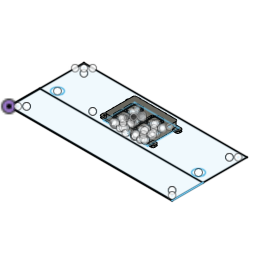
rockclimbingwall v6 (Autodesk Fusion 360 design; units mm, degrees)
Autodesk Fusion 360 part; units mm, degrees
note: some values were not read from the file. Set by a fixed rule: which sketch regions a step uses.
(part 1 of 4)
sketch "Sketch1" plane through (0, 0, 0) normal (0, 0, 1) x (1, 0, 0)
  line L0 (0, 0) -> (469.9, 0)
  line L1 (469.9, 0) -> (469.9, 215.9)
  line L2 (469.9, 215.9) -> (0, 215.9)
  line L3 (0, 215.9) -> (0, 0)
  line L4 (0, 0) -> (469.9, 0)
  line L5 (469.9, 0) -> (469.9, 88.9)
  line L6 (469.9, 88.9) -> (0, 88.9)
  line L7 (0, 88.9) -> (0, 0)
  circle A0 centre (31.75, 107.95) radius 13.97
  circle A1 centre (438.15, 107.95) radius 13.97
  circle A2 centre (234.95, 107.95) radius 3.175
  line L8 (195.58, 163.3039) -> (195.58, 144.036)
  line L9 (215.9, 144.0361) -> (215.9, 163.3039)
  line L10 (197.3761, 165.1) -> (214.104, 165.1)
  line L11 (214.104, 142.24) -> (197.3761, 142.24)
  line L12 (223.52, 163.304) -> (223.52, 144.0362)
  line L13 (187.96, 144.036) -> (187.96, 163.3039)
  line L14 (214.104, 172.72) -> (197.3761, 172.72)
  line L15 (197.3761, 134.62) -> (214.104, 134.62)
  line L16 (193.938, 168.012) -> (196.478, 165.472)
  line L17 (192.668, 166.742) -> (195.208, 164.202)
  line L18 (215.002, 165.472) -> (217.542, 168.012)
  line L19 (216.272, 164.202) -> (218.812, 166.742)
  line L20 (215.002, 172.348) -> (217.542, 169.808)
  line L21 (223.148, 164.202) -> (220.608, 166.742)
  line L22 (196.478, 172.348) -> (193.938, 169.808)
  line L23 (190.872, 166.742) -> (188.332, 164.202)
  line L24 (190.872, 140.598) -> (188.332, 143.138)
  line L25 (196.478, 134.992) -> (193.938, 137.532)
  line L26 (220.608, 140.5981) -> (223.148, 143.1381)
  line L27 (215.002, 134.992) -> (217.542, 137.532)
  line L28 (195.208, 143.138) -> (192.668, 140.598)
  line L29 (196.478, 141.868) -> (193.938, 139.328)
  line L30 (195.58, 163.83) -> (195.58, 163.83)
  line L31 (192.668, 166.742) -> (195.208, 164.202) construction
  line L32 (216.272, 143.1381) -> (218.8119, 140.5981) construction
  line L33 (214.63, 162.56) -> (214.63, 162.56)
  line L34 (218.812, 166.742) -> (216.272, 164.202) construction
  line L35 (195.208, 143.138) -> (192.668, 140.598) construction
  line L36 (216.272, 143.1381) -> (218.8119, 140.5981)
  line L37 (215.002, 141.868) -> (217.542, 139.328)
  arc A3 (197.3761, 172.72) -> (196.478, 172.348) centre (197.3761, 171.45) ccw
  arc A4 (193.938, 169.808) -> (193.938, 168.012) centre (194.8361, 168.91) ccw
  arc A5 (196.478, 165.472) -> (197.3761, 165.1) centre (197.3761, 166.37) ccw
  arc A6 (215.002, 172.348) -> (214.104, 172.72) centre (214.104, 171.45) ccw
  arc A7 (217.542, 168.012) -> (217.542, 169.808) centre (216.644, 168.91) ccw
  arc A8 (214.104, 165.1) -> (215.002, 165.472) centre (214.104, 166.37) ccw
  arc A9 (192.668, 166.742) -> (190.872, 166.742) centre (191.77, 165.844) ccw
  arc A10 (195.58, 163.3039) -> (195.208, 164.202) centre (194.31, 163.3039) ccw
  arc A11 (188.332, 164.202) -> (187.96, 163.3039) centre (189.23, 163.3039) ccw
  arc A12 (187.96, 144.036) -> (188.332, 143.138) centre (189.23, 144.036) ccw
  arc A13 (190.872, 140.598) -> (192.668, 140.598) centre (191.77, 141.496) ccw
  arc A14 (195.208, 143.138) -> (195.58, 144.036) centre (194.31, 144.036) ccw
  arc A15 (218.8119, 140.5981) -> (220.608, 140.5981) centre (219.71, 141.4962) ccw
  arc A16 (215.9, 144.0361) -> (216.272, 143.1381) centre (217.17, 144.0361) ccw
  arc A17 (223.148, 143.1381) -> (223.52, 144.0362) centre (222.25, 144.0362) ccw
  arc A18 (220.608, 166.742) -> (218.812, 166.742) centre (219.71, 165.8439) ccw
  arc A19 (223.52, 163.304) -> (223.148, 164.202) centre (222.25, 163.304) ccw
  arc A20 (216.272, 164.202) -> (215.9, 163.3039) centre (217.17, 163.3039) ccw
  arc A21 (193.938, 139.328) -> (193.938, 137.532) centre (194.8361, 138.43) ccw
  arc A22 (197.3761, 142.24) -> (196.478, 141.868) centre (197.3761, 140.97) ccw
  arc A23 (196.478, 134.992) -> (197.3761, 134.62) centre (197.3761, 135.89) ccw
  arc A24 (214.104, 134.62) -> (215.002, 134.992) centre (214.104, 135.89) ccw
  arc A25 (217.542, 137.532) -> (217.542, 139.328) centre (216.644, 138.43) ccw
  arc A26 (215.002, 141.868) -> (214.104, 142.24) centre (214.104, 140.97) ccw
  line L38 (223.148, 112.658) -> (220.608, 110.118)
  line L39 (190.872, 110.118) -> (188.332, 112.658)
  line L40 (215.002, 104.512) -> (217.542, 107.052)
  line L41 (223.52, 113.556) -> (223.52, 132.8238)
  line L42 (218.812, 110.118) -> (218.44, 110.49) construction
  line L43 (192.668, 110.118) -> (195.208, 112.658) construction
  line L44 (192.668, 110.118) -> (195.208, 112.658)
  line L45 (216.272, 112.658) -> (218.812, 110.118)
  line L46 (215.002, 111.388) -> (217.542, 108.848)
  line L47 (215.9, 132.8239) -> (215.9, 113.5561)
  line L48 (193.938, 108.848) -> (196.478, 111.388)
  arc A27 (195.208, 112.658) -> (195.58, 113.5561) centre (194.31, 113.5561) ccw
  line L49 (214.63, 114.3) -> (214.63, 114.3)
  arc A28 (214.104, 104.14) -> (215.002, 104.512) centre (214.104, 105.41) ccw
  arc A29 (190.872, 110.118) -> (192.668, 110.118) centre (191.77, 111.016) ccw
  line L50 (187.96, 132.824) -> (187.96, 113.5561)
  line L51 (197.3761, 111.76) -> (214.104, 111.76)
  line L52 (214.104, 104.14) -> (197.3761, 104.14)
  line L53 (195.58, 113.5561) -> (195.58, 132.824)
  arc A30 (223.148, 112.658) -> (223.52, 113.556) centre (222.25, 113.556) ccw
  arc A31 (215.002, 111.388) -> (214.104, 111.76) centre (214.104, 110.49) ccw
  line L54 (195.58, 113.03) -> (195.58, 113.03)
  arc A32 (196.478, 104.512) -> (197.3761, 104.14) centre (197.3761, 105.41) ccw
  arc A33 (197.3761, 111.76) -> (196.478, 111.388) centre (197.3761, 110.49) ccw
  arc A34 (215.9, 113.5561) -> (216.272, 112.658) centre (217.17, 113.5561) ccw
  line L55 (196.478, 104.512) -> (193.938, 107.052)
  arc A35 (195.58, 132.824) -> (195.208, 133.722) centre (194.31, 132.824) ccw
  arc A36 (218.812, 110.118) -> (220.608, 110.118) centre (219.71, 111.0161) ccw
  arc A37 (193.938, 108.848) -> (193.938, 107.052) centre (194.8361, 107.95) ccw
  arc A38 (187.96, 113.5561) -> (188.332, 112.658) centre (189.23, 113.5561) ccw
  arc A39 (192.668, 136.262) -> (190.872, 136.262) centre (191.77, 135.364) ccw
  line L56 (195.208, 133.722) -> (192.668, 136.262) construction
  arc A40 (223.52, 132.8238) -> (223.148, 133.7219) centre (222.25, 132.8238) ccw
  arc A41 (188.332, 133.722) -> (187.96, 132.824) centre (189.23, 132.824) ccw
  line L57 (220.608, 136.2619) -> (223.148, 133.7219)
  arc A42 (216.272, 133.7219) -> (215.9, 132.8239) centre (217.17, 132.8239) ccw
  arc A43 (220.608, 136.2619) -> (218.8119, 136.2619) centre (219.71, 135.3638) ccw
  line L58 (195.208, 133.722) -> (192.668, 136.262)
  line L59 (216.272, 133.7219) -> (218.8119, 136.2619)
  line L60 (190.872, 136.262) -> (188.332, 133.722)
  line L61 (216.272, 133.7219) -> (218.8119, 136.2619) construction
  arc A44 (217.542, 107.052) -> (217.542, 108.848) centre (216.644, 107.95) ccw
  line L62 (249.292, 136.2619) -> (246.752, 133.7219)
  arc A45 (254.898, 134.992) -> (255.796, 134.62) centre (255.796, 135.89) ccw
  line L63 (254.898, 104.512) -> (252.358, 107.052)
  line L64 (273.422, 104.512) -> (275.962, 107.052)
  line L65 (246.752, 112.658) -> (249.292, 110.118)
  line L66 (281.94, 132.824) -> (281.94, 113.5561)
  line L67 (246.38, 113.556) -> (246.38, 132.8238)
  line L68 (255.796, 104.14) -> (272.5239, 104.14)
  line L69 (279.028, 110.118) -> (281.568, 112.658)
  arc A46 (252.358, 108.848) -> (252.358, 107.052) centre (253.256, 107.95) ccw
  line L70 (277.232, 110.118) -> (274.692, 112.658)
  line L71 (253.628, 164.202) -> (251.088, 166.742)
  arc A47 (253.628, 112.658) -> (254, 113.5561) centre (252.73, 113.5561) ccw
  line L72 (254.898, 165.472) -> (252.358, 168.012)
  line L73 (275.962, 108.848) -> (273.422, 111.388)
  line L74 (274.32, 113.03) -> (274.32, 113.03)
  line L75 (272.5239, 134.62) -> (255.796, 134.62)
  arc A48 (254.898, 104.512) -> (255.796, 104.14) centre (255.796, 105.41) ccw
  arc A49 (274.692, 133.722) -> (274.32, 132.824) centre (275.59, 132.824) ccw
  arc A50 (272.5239, 104.14) -> (273.422, 104.512) centre (272.5239, 105.41) ccw
  line L76 (251.088, 110.118) -> (253.628, 112.658) construction
  line L77 (277.232, 166.742) -> (274.692, 164.202) construction
  arc A51 (246.38, 113.556) -> (246.752, 112.658) centre (247.65, 113.556) ccw
  arc A52 (275.962, 107.052) -> (275.962, 108.848) centre (275.0639, 107.95) ccw
  arc A53 (277.232, 110.118) -> (279.028, 110.118) centre (278.13, 111.016) ccw
  line L78 (255.27, 114.3) -> (255.27, 114.3)
  line L79 (277.232, 166.742) -> (274.692, 164.202)
  arc A54 (274.32, 113.5561) -> (274.692, 112.658) centre (275.59, 113.5561) ccw
  line L80 (254, 132.8239) -> (254, 113.5561)
  arc A55 (281.94, 132.824) -> (281.568, 133.722) centre (280.67, 132.824) ccw
  line L81 (274.32, 113.5561) -> (274.32, 132.824)
  arc A56 (255.796, 111.76) -> (254.898, 111.388) centre (255.796, 110.49) ccw
  arc A57 (281.568, 112.658) -> (281.94, 113.5561) centre (280.67, 113.5561) ccw
  line L82 (253.628, 133.7219) -> (251.0881, 136.2619)
  line L83 (279.028, 136.262) -> (281.568, 133.722)
  line L84 (253.628, 133.7219) -> (251.0881, 136.2619) construction
  arc A58 (249.292, 110.118) -> (251.088, 110.118) centre (250.19, 111.0161) ccw
  line L85 (274.692, 133.722) -> (277.232, 136.262) construction
  line L86 (274.692, 133.722) -> (277.232, 136.262)
  arc A59 (246.752, 133.7219) -> (246.38, 132.8238) centre (247.65, 132.8238) ccw
  line L87 (254.898, 111.388) -> (252.358, 108.848)
  arc A60 (272.5239, 134.62) -> (273.422, 134.992) centre (272.5239, 135.89) ccw
  line L88 (253.628, 112.658) -> (251.088, 110.118)
  arc A61 (273.422, 111.388) -> (272.5239, 111.76) centre (272.5239, 110.49) ccw
  line L89 (251.088, 166.742) -> (253.628, 164.202) construction
  arc A62 (255.796, 172.72) -> (254.898, 172.348) centre (255.796, 171.45) ccw
  line L90 (255.27, 162.56) -> (255.27, 162.56)
  arc A63 (246.38, 144.0362) -> (246.752, 143.1381) centre (247.65, 144.0362) ccw
  line L91 (272.5239, 111.76) -> (255.796, 111.76)
  arc A64 (279.028, 166.742) -> (277.232, 166.742) centre (278.13, 165.844) ccw
  line L92 (274.32, 163.3039) -> (274.32, 144.036)
  line L93 (281.94, 144.036) -> (281.94, 163.3039)
  arc A65 (275.962, 168.012) -> (275.962, 169.808) centre (275.0639, 168.91) ccw
  line L94 (255.796, 172.72) -> (272.5239, 172.72)
  line L95 (253.628, 143.1381) -> (251.0881, 140.5981) construction
  line L96 (272.5239, 165.1) -> (255.796, 165.1)
  line L97 (277.232, 110.118) -> (274.692, 112.658) construction
  arc A66 (252.358, 169.808) -> (252.358, 168.012) centre (253.256, 168.91) ccw
  line L98 (246.752, 164.202) -> (249.292, 166.742)
  line L99 (254.898, 172.348) -> (252.358, 169.808)
  arc A67 (272.5239, 165.1) -> (273.422, 165.472) centre (272.5239, 166.37) ccw
  line L100 (246.38, 163.304) -> (246.38, 144.0362)
  line L101 (273.422, 141.868) -> (275.962, 139.328)
  line L102 (255.796, 142.24) -> (272.5239, 142.24)
  line L103 (279.028, 140.598) -> (281.568, 143.138)
  arc A68 (249.292, 140.5981) -> (251.0881, 140.5981) centre (250.19, 141.4962) ccw
  line L104 (273.422, 134.992) -> (275.962, 137.532)
  arc A69 (281.94, 163.3039) -> (281.568, 164.202) centre (280.67, 163.3039) ccw
  arc A70 (252.358, 139.328) -> (252.358, 137.532) centre (253.256, 138.43) ccw
  arc A71 (254, 163.3039) -> (253.628, 164.202) centre (252.73, 163.3039) ccw
  line L105 (274.32, 163.83) -> (274.32, 163.83)
  arc A72 (251.088, 166.742) -> (249.292, 166.742) centre (250.19, 165.8439) ccw
  line L106 (274.692, 143.138) -> (277.232, 140.598) construction
  line L107 (274.692, 143.138) -> (277.232, 140.598)
  line L108 (254.898, 141.868) -> (252.358, 139.328)
  line L109 (253.628, 143.1381) -> (251.0881, 140.5981)
  line L110 (273.422, 172.348) -> (275.962, 169.808)
  arc A73 (254.898, 165.472) -> (255.796, 165.1) centre (255.796, 166.37) ccw
  line L111 (275.962, 168.012) -> (273.422, 165.472)
  line L112 (279.028, 166.742) -> (281.568, 164.202)
  line L113 (254, 144.0361) -> (254, 163.3039)
  arc A74 (255.796, 142.24) -> (254.898, 141.868) centre (255.796, 140.97) ccw
  arc A75 (273.422, 172.348) -> (272.5239, 172.72) centre (272.5239, 171.45) ccw
  arc A76 (253.628, 143.1381) -> (254, 144.0361) centre (252.73, 144.0361) ccw
  line L114 (249.292, 140.5981) -> (246.752, 143.1381)
  arc A77 (246.752, 164.202) -> (246.38, 163.304) centre (247.65, 163.304) ccw
  line L115 (254.898, 134.992) -> (252.358, 137.532)
  arc A78 (275.962, 137.532) -> (275.962, 139.328) centre (275.0639, 138.43) ccw
  arc A79 (274.692, 164.202) -> (274.32, 163.3039) centre (275.59, 163.3039) ccw
  arc A80 (273.422, 141.868) -> (272.5239, 142.24) centre (272.5239, 140.97) ccw
  arc A81 (281.568, 143.138) -> (281.94, 144.036) centre (280.67, 144.036) ccw
  arc A82 (279.028, 136.262) -> (277.232, 136.262) centre (278.13, 135.364) ccw
  arc A83 (251.0881, 136.2619) -> (249.292, 136.2619) centre (250.19, 135.3638) ccw
  arc A84 (274.32, 144.036) -> (274.692, 143.138) centre (275.59, 144.036) ccw
  arc A85 (277.232, 140.598) -> (279.028, 140.598) centre (278.13, 141.496) ccw
  arc A86 (254, 132.8239) -> (253.628, 133.7219) centre (252.73, 132.8239) ccw
  line L116 (234.95, 101.6) -> (298.45, 101.6)
  line L117 (298.45, 101.6) -> (171.45, 101.6)
  line L118 (171.45, 101.6) -> (171.45, 190.5)
  line L119 (171.45, 190.5) -> (298.45, 190.5)
  line L120 (298.45, 190.5) -> (298.45, 101.6)
  circle A87 centre (189.23, 110.49) radius 1.5875
  circle A88 centre (281.94, 110.49) radius 1.5875
  circle A89 centre (281.94, 180.34) radius 1.5875
  circle A90 centre (189.23, 180.34) radius 1.5875
  circle A91 centre (133.35, 107.95) radius 3.175
  circle A92 centre (133.35, 107.95) radius 6.35
  line L121 (281.94, 113.5561) -> (281.94, 132.824)
  line L122 (281.94, 144.036) -> (281.94, 163.3039)
  line L123 (0, 215.9) -> (25.4, 215.9)
  line L124 (0, 190.5) -> (0, 215.9)
  circle A93 centre (25.4, 190.5) radius 6.35
  circle A94 centre (444.5, 190.5) radius 6.35
  circle A95 centre (25.4, 25.4) radius 6.35
  circle A96 centre (444.5, 25.4) radius 6.35
  circle A97 centre (25.4, 190.5) radius 4.1275
  line L125 (171.45, 190.5) -> (298.45, 190.5)
  circle A98 centre (444.5, 190.5) radius 4.1275
  circle A99 centre (444.5, 25.4) radius 4.1275
  circle A100 centre (25.4, 25.4) radius 4.1275
  circle A101 centre (12.7, 203.2) radius 0.635
  circle A102 centre (457.2, 203.2) radius 0.635
  circle A103 centre (457.2, 12.7) radius 0.635
  circle A104 centre (12.7, 12.7) radius 0.635
  point P0 (214.63, 165.1)
  point P1 (214.63, 142.24)
  point P2 (196.85, 142.24)
  point P3 (205.74, 153.67)
  point P4 (205.74, 153.67)
  point P5 (205.74, 153.67)
  point P6 (214.104, 134.62)
  point P7 (215.002, 134.992)
  point P8 (214.63, 111.76)
  point P9 (197.3761, 134.62)
  point P10 (214.63, 134.62)
  point P11 (196.478, 134.992)
  point P12 (191.77, 115.57)
  point P13 (213.36, 107.95)
  point P14 (214.104, 135.89)
  point P15 (219.71, 130.81)
  point P16 (219.71, 115.57)
  point P17 (197.3761, 135.89)
  point P18 (205.74, 123.19)
  point P19 (205.74, 123.19)
  point P20 (196.85, 134.62)
  point P21 (198.12, 107.95)
  point P22 (205.74, 123.19)
  point P23 (191.77, 130.81)
  point P24 (264.16, 153.67)
  point P25 (264.16, 123.19)
  point P26 (264.16, 123.19)
  point P27 (278.13, 130.81)
  point P28 (255.796, 135.89)
  point P29 (254.898, 134.992)
  point P30 (273.422, 134.992)
  point P31 (255.27, 142.24)
  point P32 (255.27, 165.1)
  point P33 (278.13, 115.57)
  point P34 (255.27, 134.62)
  point P35 (273.05, 134.62)
  point P36 (264.16, 153.67)
  point P37 (255.27, 111.76)
  point P38 (250.19, 130.81)
  point P39 (256.54, 107.95)
  point P40 (264.16, 153.67)
  point P41 (272.5239, 135.89)
  point P42 (272.5239, 134.62)
  point P43 (256.54, 107.95)
  point P44 (250.19, 115.57)
  point P45 (271.78, 107.95)
  point P46 (273.05, 142.24)
  point P47 (255.796, 134.62)
  point P48 (264.16, 123.19)
  dimension "d1" = 469.9
  dimension "d2" = 215.9
  dimension "d3" = 88.9
  dimension "d5" = 27.94
  dimension "d7" = 27.94
  dimension "d9" = 6.35
  dimension "d37" = 17.78
  dimension "d38" = 22.86
  dimension "d42" = 1.27
  dimension "d43" = 63.5
  dimension "d44" = 127
  dimension "d45" = 88.9
  dimension "d48" = 3.175
  dimension "d49" = 69.85
  dimension "d50" = 3.175
  dimension "d51" = 3.175
  dimension "d52" = 3.175
  dimension "d53" = 101.6
  dimension "d54" = 6.35
  dimension "d55" = 12.7
  dimension "d56" = 12.7
  dimension "d57" = 12.7
  dimension "d58" = 12.7
  dimension "d59" = 12.7
  dimension "d60" = 8.255
  dimension "d61" = 8.255
  dimension "d62" = 8.255
  dimension "d63" = 8.255
  dimension "d64" = 1.27
  dimension "d65" = 1.27
  dimension "d66" = 1.27
  dimension "d67" = 1.27
  constraint horizontal L0
  constraint vertical L1
  constraint horizontal L2
  constraint vertical L3
  constraint coincident L0.start L3.end
  constraint horizontal L4
  constraint vertical L5
  constraint horizontal L6
  constraint vertical L7
  constraint parallel L8 L9
  constraint horizontal L10
  constraint parallel L10 L11
  constraint parallel L12 L13
  constraint coincident P5 L31
  constraint coincident P5 L34
  constraint coincident P5 P4
  constraint horizontal L14
  constraint parallel L14 L15
  constraint perpendicular L23 L24
  constraint perpendicular L26 L36
  constraint collinear L31 L32
  constraint collinear L34 L35
  constraint tangent L22 A3
  constraint tangent L14 A3
  constraint tangent L22 A4
  constraint tangent L16 A4
  constraint equal A3 A4
  constraint tangent L10 A5
  constraint tangent L16 A5
  constraint equal A3 A5
  constraint tangent L20 A6
  constraint tangent L14 A6
  constraint equal A3 A6
  constraint tangent L20 A7
  constraint tangent L18 A7
  constraint equal A3 A7
  constraint coincident P0 L10
  constraint coincident P0 L18
  constraint tangent L10 A8
  constraint tangent L18 A8
  constraint equal A3 A8
  constraint tangent L31 A9
  constraint tangent L23 A9
  constraint equal A3 A9
  constraint coincident L30.start L31
  constraint coincident L30.start L8
  constraint tangent L31 A10
  constraint tangent L8 A10
  constraint equal A3 A10
  constraint tangent L13 A11
  constraint tangent L23 A11
  constraint equal A3 A11
  constraint tangent L13 A12
  constraint tangent L24 A12
  constraint equal A3 A12
  constraint tangent L28 A13
  constraint tangent L24 A13
  constraint equal A3 A13
  constraint tangent L28 A14
  constraint tangent L8 A14
  constraint equal A3 A14
  constraint tangent L32 A15
  constraint tangent L26 A15
  constraint equal A3 A15
  constraint tangent L36 A16
  constraint tangent L9 A16
  constraint equal A3 A16
  constraint tangent L26 A17
  constraint tangent L12 A17
  constraint equal A3 A17
  constraint tangent L34 A18
  constraint tangent L21 A18
  constraint equal A3 A18
  constraint tangent L21 A19
  constraint tangent L12 A19
  constraint equal A3 A19
  constraint tangent L9 A20
  constraint tangent L19 A20
  constraint equal A3 A20
  constraint tangent L29 A21
  constraint tangent L25 A21
  constraint equal A3 A21
  constraint coincident P2 L29
  constraint coincident P2 L11
  constraint tangent L29 A22
  constraint tangent L11 A22
  constraint equal A3 A22
  constraint tangent L25 A23
  constraint tangent L15 A23
  constraint equal A3 A23
  constraint tangent L15 A24
  constraint tangent L27 A24
  constraint equal A3 A24
  constraint tangent L37 A25
  constraint tangent L27 A25
  constraint equal A3 A25
  constraint coincident P1 L11
  constraint coincident P1 L37
  constraint tangent L11 A26
  constraint tangent L37 A26
  constraint equal A3 A26
  constraint horizontal L117
  constraint vertical L118
  constraint horizontal L119
  constraint vertical L120
  constraint vertical L121
  constraint concentric A91 A92
  constraint collinear L121 L122
  constraint horizontal L123
  constraint vertical L124
  constraint horizontal L125
  constraint concentric A93 A97
  constraint concentric A94 A98
  constraint concentric A96 A99
  constraint concentric A95 A100
  measures "d1" distance of L0.start L0.end
  measures "d2" distance of L0.start L2.end
  measures "d3" distance of L0.start L6.end
  measures "d5" diameter of A0
  measures "d7" diameter of A1
  measures "d9" diameter of A2
  measures "d37" distance of P1 P2
  measures "d38" distance of P0 P1
  measures "d42" radius of A3
  measures "d43" distance of L116.start L116.end
  measures "d44" distance of L116.end L117.end
  measures "d45" distance of L116.end L119.end
  measures "d48" diameter of A87
  measures "d49" distance of A87.centre A90.centre
  measures "d50" diameter of A88
  measures "d51" diameter of A89
  measures "d52" diameter of A90
  measures "d53" distance of A2.centre A91.centre
  measures "d54" diameter of A91
  measures "d55" diameter of A92
  measures "d56" diameter of A93
  measures "d57" diameter of A94
  measures "d58" diameter of A95
  measures "d59" diameter of A96
  measures "d60" diameter of A97
  measures "d61" diameter of A98
  measures "d62" diameter of A99
  measures "d63" diameter of A100
  measures "d64" diameter of A101
  measures "d65" diameter of A102
  measures "d66" diameter of A103
  measures "d67" diameter of A104
extrude "Extrude1" add sketch "Sketch1" along normal blind 25.4 contours L0 L1 L3 L4 L5 L6 L7 | L1 L2 L3 L6 L123 L124 | L39 A87 | L116 L117 L118 L119 L120 L125 | A88 | A89 | A90 | A92 | A93 | A94 | A95 | A96 picked at (189.0956, 109.9792) makes body 1
sketch "Sketch2" plane through (0, 0, 25.4) normal (0, 0, 1) x (-1, 0, 0)
  arc A0 (-196.478, -134.992) -> (-197.3761, -134.62) centre (-197.3761, -135.89) ccw
  line L0 (-196.478, -134.992) -> (-193.938, -137.532)
  arc A1 (-193.938, -139.328) -> (-193.938, -137.532) centre (-194.8361, -138.43) ccw
  line L1 (-193.938, -139.328) -> (-196.478, -141.868)
  arc A2 (-197.3761, -142.24) -> (-196.478, -141.868) centre (-197.3761, -140.97) ccw
  line L2 (-197.3761, -142.24) -> (-214.104, -142.24)
  arc A3 (-215.002, -141.868) -> (-214.104, -142.24) centre (-214.104, -140.97) ccw
  line L3 (-215.002, -141.868) -> (-217.542, -139.328)
  arc A4 (-217.542, -137.532) -> (-217.542, -139.328) centre (-216.644, -138.43) ccw
  line L4 (-217.542, -137.532) -> (-215.002, -134.992)
  arc A5 (-214.104, -134.62) -> (-215.002, -134.992) centre (-214.104, -135.89) ccw
  line L5 (-214.104, -134.62) -> (-197.3761, -134.62)
  arc A6 (-223.52, -163.304) -> (-223.148, -164.202) centre (-222.25, -163.304) ccw
  line L6 (-223.52, -163.304) -> (-223.52, -144.0362)
  arc A7 (-223.148, -143.1381) -> (-223.52, -144.0362) centre (-222.25, -144.0362) ccw
  line L7 (-223.148, -143.1381) -> (-220.608, -140.5981)
  arc A8 (-218.8119, -140.5981) -> (-220.608, -140.5981) centre (-219.71, -141.4962) ccw
  line L8 (-218.8119, -140.5981) -> (-216.272, -143.1381)
  arc A9 (-215.9, -144.0361) -> (-216.272, -143.1381) centre (-217.17, -144.0361) ccw
  line L9 (-215.9, -144.0361) -> (-215.9, -163.3039)
  arc A10 (-216.272, -164.202) -> (-215.9, -163.3039) centre (-217.17, -163.3039) ccw
  line L10 (-216.272, -164.202) -> (-218.812, -166.742)
  arc A11 (-220.608, -166.742) -> (-218.812, -166.742) centre (-219.71, -165.8439) ccw
  line L11 (-220.608, -166.742) -> (-223.148, -164.202)
  arc A12 (-215.002, -172.348) -> (-214.104, -172.72) centre (-214.104, -171.45) ccw
  line L12 (-215.002, -172.348) -> (-217.542, -169.808)
  arc A13 (-217.542, -168.012) -> (-217.542, -169.808) centre (-216.644, -168.91) ccw
  line L13 (-217.542, -168.012) -> (-215.002, -165.472)
  arc A14 (-214.104, -165.1) -> (-215.002, -165.472) centre (-214.104, -166.37) ccw
  line L14 (-214.104, -165.1) -> (-197.3761, -165.1)
  arc A15 (-196.478, -165.472) -> (-197.3761, -165.1) centre (-197.3761, -166.37) ccw
  line L15 (-196.478, -165.472) -> (-193.938, -168.012)
  arc A16 (-193.938, -169.808) -> (-193.938, -168.012) centre (-194.8361, -168.91) ccw
  line L16 (-193.938, -169.808) -> (-196.478, -172.348)
  arc A17 (-197.3761, -172.72) -> (-196.478, -172.348) centre (-197.3761, -171.45) ccw
  line L17 (-197.3761, -172.72) -> (-214.104, -172.72)
  arc A18 (-190.872, -140.598) -> (-192.668, -140.598) centre (-191.77, -141.496) ccw
  line L18 (-190.872, -140.598) -> (-188.332, -143.138)
  arc A19 (-187.96, -144.036) -> (-188.332, -143.138) centre (-189.23, -144.036) ccw
  line L19 (-187.96, -144.036) -> (-187.96, -163.3039)
  arc A20 (-188.332, -164.202) -> (-187.96, -163.3039) centre (-189.23, -163.3039) ccw
  line L20 (-188.332, -164.202) -> (-190.872, -166.742)
  arc A21 (-192.668, -166.742) -> (-190.872, -166.742) centre (-191.77, -165.844) ccw
  line L21 (-192.668, -166.742) -> (-195.208, -164.202)
  arc A22 (-195.58, -163.3039) -> (-195.208, -164.202) centre (-194.31, -163.3039) ccw
  line L22 (-195.58, -163.3039) -> (-195.58, -144.036)
  arc A23 (-195.208, -143.138) -> (-195.58, -144.036) centre (-194.31, -144.036) ccw
  line L23 (-195.208, -143.138) -> (-192.668, -140.598)
  circle A24 centre (-234.95, -107.95) radius 3.175
  circle A25 centre (-25.4, -190.5) radius 4.1275
  circle A26 centre (-444.5, -190.5) radius 4.1275
  circle A27 centre (-12.7, -12.7) radius 0.635
  arc A28 (-254.898, -104.512) -> (-255.796, -104.14) centre (-255.796, -105.41) ccw
  line L24 (-254.898, -104.512) -> (-252.358, -107.052)
  arc A29 (-252.358, -108.848) -> (-252.358, -107.052) centre (-253.256, -107.95) ccw
  line L25 (-252.358, -108.848) -> (-254.898, -111.388)
  arc A30 (-255.796, -111.76) -> (-254.898, -111.388) centre (-255.796, -110.49) ccw
  line L26 (-255.796, -111.76) -> (-272.5239, -111.76)
  arc A31 (-273.422, -111.388) -> (-272.5239, -111.76) centre (-272.5239, -110.49) ccw
  line L27 (-273.422, -111.388) -> (-275.962, -108.848)
  arc A32 (-275.962, -107.052) -> (-275.962, -108.848) centre (-275.0639, -107.95) ccw
  line L28 (-275.962, -107.052) -> (-273.422, -104.512)
  arc A33 (-272.5239, -104.14) -> (-273.422, -104.512) centre (-272.5239, -105.41) ccw
  line L29 (-272.5239, -104.14) -> (-255.796, -104.14)
  circle A34 centre (-25.4, -25.4) radius 4.1275
  arc A35 (-275.962, -168.012) -> (-275.962, -169.808) centre (-275.0639, -168.91) ccw
  line L30 (-275.962, -168.012) -> (-273.422, -165.472)
  arc A36 (-272.5239, -165.1) -> (-273.422, -165.472) centre (-272.5239, -166.37) ccw
  line L31 (-272.5239, -165.1) -> (-255.796, -165.1)
  arc A37 (-254.898, -165.472) -> (-255.796, -165.1) centre (-255.796, -166.37) ccw
  line L32 (-254.898, -165.472) -> (-252.358, -168.012)
  arc A38 (-252.358, -169.808) -> (-252.358, -168.012) centre (-253.256, -168.91) ccw
  line L33 (-252.358, -169.808) -> (-254.898, -172.348)
  arc A39 (-255.796, -172.72) -> (-254.898, -172.348) centre (-255.796, -171.45) ccw
  line L34 (-255.796, -172.72) -> (-272.5239, -172.72)
  arc A40 (-273.422, -172.348) -> (-272.5239, -172.72) centre (-272.5239, -171.45) ccw
  line L35 (-273.422, -172.348) -> (-275.962, -169.808)
  circle A41 centre (-457.2, -12.7) radius 0.635
  arc A42 (-253.628, -143.1381) -> (-254, -144.0361) centre (-252.73, -144.0361) ccw
  line L36 (-253.628, -143.1381) -> (-251.0881, -140.5981)
  arc A43 (-249.292, -140.5981) -> (-251.0881, -140.5981) centre (-250.19, -141.4962) ccw
  line L37 (-249.292, -140.5981) -> (-246.752, -143.1381)
  arc A44 (-246.38, -144.0362) -> (-246.752, -143.1381) centre (-247.65, -144.0362) ccw
  line L38 (-246.38, -144.0362) -> (-246.38, -163.304)
  arc A45 (-246.752, -164.202) -> (-246.38, -163.304) centre (-247.65, -163.304) ccw
  line L39 (-246.752, -164.202) -> (-249.292, -166.742)
  arc A46 (-251.088, -166.742) -> (-249.292, -166.742) centre (-250.19, -165.8439) ccw
  line L40 (-251.088, -166.742) -> (-253.628, -164.202)
  arc A47 (-254, -163.3039) -> (-253.628, -164.202) centre (-252.73, -163.3039) ccw
  line L41 (-254, -163.3039) -> (-254, -144.0361)
  arc A48 (-272.5239, -134.62) -> (-273.422, -134.992) centre (-272.5239, -135.89) ccw
  line L42 (-272.5239, -134.62) -> (-255.796, -134.62)
  arc A49 (-254.898, -134.992) -> (-255.796, -134.62) centre (-255.796, -135.89) ccw
  line L43 (-254.898, -134.992) -> (-252.358, -137.532)
  arc A50 (-252.358, -139.328) -> (-252.358, -137.532) centre (-253.256, -138.43) ccw
  line L44 (-252.358, -139.328) -> (-254.898, -141.868)
  arc A51 (-255.796, -142.24) -> (-254.898, -141.868) centre (-255.796, -140.97) ccw
  line L45 (-255.796, -142.24) -> (-272.5239, -142.24)
  arc A52 (-273.422, -141.868) -> (-272.5239, -142.24) centre (-272.5239, -140.97) ccw
  line L46 (-273.422, -141.868) -> (-275.962, -139.328)
  arc A53 (-275.962, -137.532) -> (-275.962, -139.328) centre (-275.0639, -138.43) ccw
  line L47 (-275.962, -137.532) -> (-273.422, -134.992)
  circle A54 centre (-457.2, -203.2) radius 0.635
  circle A55 centre (-133.35, -107.95) radius 3.175
  arc A56 (-253.628, -112.658) -> (-254, -113.5561) centre (-252.73, -113.5561) ccw
  line L48 (-253.628, -112.658) -> (-251.088, -110.118)
  arc A57 (-249.292, -110.118) -> (-251.088, -110.118) centre (-250.19, -111.0161) ccw
  line L49 (-249.292, -110.118) -> (-246.752, -112.658)
  arc A58 (-246.38, -113.556) -> (-246.752, -112.658) centre (-247.65, -113.556) ccw
  line L50 (-246.38, -113.556) -> (-246.38, -132.8238)
  arc A59 (-246.752, -133.7219) -> (-246.38, -132.8238) centre (-247.65, -132.8238) ccw
  line L51 (-246.752, -133.7219) -> (-249.292, -136.2619)
  arc A60 (-251.0881, -136.2619) -> (-249.292, -136.2619) centre (-250.19, -135.3638) ccw
  line L52 (-251.0881, -136.2619) -> (-253.628, -133.7219)
  arc A61 (-254, -132.8239) -> (-253.628, -133.7219) centre (-252.73, -132.8239) ccw
  line L53 (-254, -132.8239) -> (-254, -113.5561)
  arc A62 (-277.232, -110.118) -> (-279.028, -110.118) centre (-278.13, -111.016) ccw
  line L54 (-277.232, -110.118) -> (-274.692, -112.658)
  arc A63 (-274.32, -113.5561) -> (-274.692, -112.658) centre (-275.59, -113.5561) ccw
  line L55 (-274.32, -113.5561) -> (-274.32, -132.824)
  arc A64 (-274.692, -133.722) -> (-274.32, -132.824) centre (-275.59, -132.824) ccw
  line L56 (-274.692, -133.722) -> (-277.232, -136.262)
  arc A65 (-279.028, -136.262) -> (-277.232, -136.262) centre (-278.13, -135.364) ccw
  line L57 (-279.028, -136.262) -> (-281.568, -133.722)
  arc A66 (-281.94, -132.824) -> (-281.568, -133.722) centre (-280.67, -132.824) ccw
  line L58 (-281.94, -132.824) -> (-281.94, -113.5561)
  arc A67 (-281.568, -112.658) -> (-281.94, -113.5561) centre (-280.67, -113.5561) ccw
  line L59 (-281.568, -112.658) -> (-279.028, -110.118)
  circle A68 centre (-438.15, -107.95) radius 13.97
  circle A69 centre (-31.75, -107.95) radius 13.97
  circle A70 centre (-12.7, -203.2) radius 0.635
  circle A71 centre (-444.5, -25.4) radius 4.1275
  arc A72 (-279.028, -166.742) -> (-277.232, -166.742) centre (-278.13, -165.844) ccw
  line L60 (-279.028, -166.742) -> (-281.568, -164.202)
  arc A73 (-281.94, -163.3039) -> (-281.568, -164.202) centre (-280.67, -163.3039) ccw
  line L61 (-281.94, -163.3039) -> (-281.94, -144.036)
  arc A74 (-281.568, -143.138) -> (-281.94, -144.036) centre (-280.67, -144.036) ccw
  line L62 (-281.568, -143.138) -> (-279.028, -140.598)
  arc A75 (-277.232, -140.598) -> (-279.028, -140.598) centre (-278.13, -141.496) ccw
  line L63 (-277.232, -140.598) -> (-274.692, -143.138)
  arc A76 (-274.32, -144.036) -> (-274.692, -143.138) centre (-275.59, -144.036) ccw
  line L64 (-274.32, -144.036) -> (-274.32, -163.3039)
  arc A77 (-274.692, -164.202) -> (-274.32, -163.3039) centre (-275.59, -163.3039) ccw
  line L65 (-274.692, -164.202) -> (-277.232, -166.742)
  arc A78 (-214.104, -104.14) -> (-215.002, -104.512) centre (-214.104, -105.41) ccw
  line L66 (-214.104, -104.14) -> (-197.3761, -104.14)
  arc A79 (-196.478, -104.512) -> (-197.3761, -104.14) centre (-197.3761, -105.41) ccw
  line L67 (-196.478, -104.512) -> (-193.938, -107.052)
  arc A80 (-193.938, -108.848) -> (-193.938, -107.052) centre (-194.8361, -107.95) ccw
  line L68 (-193.938, -108.848) -> (-196.478, -111.388)
  arc A81 (-197.3761, -111.76) -> (-196.478, -111.388) centre (-197.3761, -110.49) ccw
  line L69 (-197.3761, -111.76) -> (-214.104, -111.76)
  arc A82 (-215.002, -111.388) -> (-214.104, -111.76) centre (-214.104, -110.49) ccw
  line L70 (-215.002, -111.388) -> (-217.542, -108.848)
  arc A83 (-217.542, -107.052) -> (-217.542, -108.848) centre (-216.644, -107.95) ccw
  line L71 (-217.542, -107.052) -> (-215.002, -104.512)
  line L72 (-215.9, -113.5561) -> (-215.9, -132.8239)
  arc A84 (-216.272, -133.7219) -> (-215.9, -132.8239) centre (-217.17, -132.8239) ccw
  line L73 (-216.272, -133.7219) -> (-218.8119, -136.2619)
  arc A85 (-220.608, -136.2619) -> (-218.8119, -136.2619) centre (-219.71, -135.3638) ccw
  line L74 (-220.608, -136.2619) -> (-223.148, -133.7219)
  arc A86 (-223.52, -132.8238) -> (-223.148, -133.7219) centre (-222.25, -132.8238) ccw
  line L75 (-223.52, -132.8238) -> (-223.52, -113.556)
  arc A87 (-223.148, -112.658) -> (-223.52, -113.556) centre (-222.25, -113.556) ccw
  line L76 (-223.148, -112.658) -> (-220.608, -110.118)
  arc A88 (-218.812, -110.118) -> (-220.608, -110.118) centre (-219.71, -111.0161) ccw
  line L77 (-218.812, -110.118) -> (-216.272, -112.658)
  arc A89 (-215.9, -113.5561) -> (-216.272, -112.658) centre (-217.17, -113.5561) ccw
  arc A90 (-190.872, -110.118) -> (-192.668, -110.118) centre (-191.77, -111.016) ccw
  line L78 (-190.872, -110.118) -> (-188.332, -112.658)
  arc A91 (-187.96, -113.5561) -> (-188.332, -112.658) centre (-189.23, -113.5561) ccw
  line L79 (-187.96, -113.5561) -> (-187.96, -132.824)
  arc A92 (-188.332, -133.722) -> (-187.96, -132.824) centre (-189.23, -132.824) ccw
  line L80 (-188.332, -133.722) -> (-190.872, -136.262)
  arc A93 (-192.668, -136.262) -> (-190.872, -136.262) centre (-191.77, -135.364) ccw
  line L81 (-192.668, -136.262) -> (-195.208, -133.722)
  arc A94 (-195.58, -132.824) -> (-195.208, -133.722) centre (-194.31, -132.824) ccw
  line L82 (-195.58, -132.824) -> (-195.58, -113.5561)
  arc A95 (-195.208, -112.658) -> (-195.58, -113.5561) centre (-194.31, -113.5561) ccw
  line L83 (-195.208, -112.658) -> (-192.668, -110.118)
  line L84 (0, -215.9) -> (0, 0)
  line L85 (0, 0) -> (-469.9, 0)
  line L86 (-469.9, 0) -> (-469.9, -215.9)
  line L87 (-469.9, -215.9) -> (0, -215.9)
  spline S0 degree 3 poles (-329.0355, 18.5722) (-326.7611, 16.8724) (-327.4338, 15.4917) (-331.9278, 12.6358) knots 0 0 0 0 1 1 1 1
  spline S1 degree 3 poles (-331.9278, 12.6358) (-333.6565, 11.5373) (-336.6388, 7.5165) (-338.555, 3.701) knots 0 0 0 0 1 1 1 1
  spline S2 degree 3 poles (-338.555, 3.701) (-340.4712, -0.1144) (-344.838, -8.5214) (-348.2586, -14.9809) knots 0 0 0 0 1 1 1 1
  spline S3 degree 3 poles (-348.2586, -14.9809) (-351.6792, -21.4404) (-354.4778, -27.5581) (-354.4778, -28.5764) knots 0 0 0 0 1 1 1 1
  spline S4 degree 3 poles (-354.4778, -28.5764) (-354.4778, -29.5947) (-356.685, -34.4266) (-359.3827, -39.3133) knots 0 0 0 0 1 1 1 1
  spline S5 degree 3 poles (-359.3827, -39.3133) (-362.0803, -44.2) (-364.097, -48.3222) (-363.8641, -48.4729) knots 0 0 0 0 1 1 1 1
  spline S6 degree 3 poles (-363.8641, -48.4729) (-356.973, -52.9332) (-354.4925, -54.769) (-354.4861, -55.414) knots 0 0 0 0 1 1 1 1
  spline S7 degree 3 poles (-354.4861, -55.414) (-354.4815, -55.8492) (-352.3092, -56.5716) (-349.6584, -57.0194) knots 0 0 0 0 1 1 1 1
  spline S8 degree 3 poles (-349.6584, -57.0194) (-346.2683, -57.5922) (-344.0393, -57.3097) (-342.1423, -56.0668) knots 0 0 0 0 1 1 1 1
  spline S9 degree 3 poles (-342.1423, -56.0668) (-340.6591, -55.095) (-334.9861, -52.7898) (-329.5358, -50.9442) knots 0 0 0 0 1 1 1 1
  spline S10 degree 3 poles (-329.5358, -50.9442) (-318.8808, -47.3363) (-315.9974, -47.6815) (-315.2579, -52.6535) knots 0 0 0 0 1 1 1 1
  spline S11 degree 3 poles (-315.2579, -52.6535) (-315.0479, -54.0652) (-314.344, -55.2202) (-313.6936, -55.2202) knots 0 0 0 0 1 1 1 1
  spline S12 degree 3 poles (-313.6936, -55.2202) (-313.0432, -55.2202) (-312.8205, -54.7196) (-313.1987, -54.1078) knots 0 0 0 0 1 1 1 1
  spline S13 degree 3 poles (-313.1987, -54.1078) (-313.5769, -53.4959) (-313.3397, -52.6576) (-312.6717, -52.2447) knots 0 0 0 0 1 1 1 1
  spline S14 degree 3 poles (-312.6717, -52.2447) (-312.0037, -51.8319) (-311.4572, -52.0085) (-311.4572, -52.6371) knots 0 0 0 0 1 1 1 1
  spline S15 degree 3 poles (-311.4572, -52.6371) (-311.4572, -53.2657) (-309.7095, -53.7008) (-307.5734, -53.6039) knots 0 0 0 0 1 1 1 1
  spline S16 degree 3 poles (-307.5734, -53.6039) (-304.1228, -53.4473) (-303.7162, -53.761) (-303.9287, -56.4153) knots 0 0 0 0 1 1 1 1
  spline S17 degree 3 poles (-303.9287, -56.4153) (-304.0603, -58.0584) (-303.8818, -61.4006) (-303.532, -63.8424) knots 0 0 0 0 1 1 1 1
  line L88 (-303.532, -63.8424) -> (-302.8961, -68.2819)
  line L89 (-302.8961, -68.2819) -> (-294.9276, -62.3044)
  spline S18 degree 3 poles (-294.9276, -62.3044) (-290.5449, -59.0168) (-282.9288, -53.2546) (-278.0022, -49.4997) knots 0 0 0 0 1 1 1 1
  spline S19 degree 3 poles (-278.0022, -49.4997) (-269.6477, -43.1315) (-249.0728, -30.1745) (-247.1739, -30.0848) knots 0 0 0 0 1 1 1 1
  spline S20 degree 3 poles (-247.1739, -30.0848) (-244.6533, -29.9662) (-241.1428, -25.4651) (-241.7525, -23.1333) knots 0 0 0 0 1 1 1 1
  spline S21 degree 3 poles (-241.7525, -23.1333) (-242.2366, -21.2822) (-241.2992, -19.5409) (-238.2871, -16.6962) knots 0 0 0 0 1 1 1 1
  spline S22 degree 3 poles (-238.2871, -16.6962) (-230.8144, -9.6389) (-227.6497, -7.419) (-217.2124, -1.9134) knots 0 0 0 0 1 1 1 1
  line L90 (-217.2124, -1.9134) -> (-213.5849, 0)
  spline S23 degree 3 poles (-454.8506, -193.8468) (-449.9333, -190.6228) (-438.1872, -177.9547) (-433.5752, -170.9019) knots 0 0 0 0 1 1 1 1
  spline S24 degree 3 poles (-433.5752, -170.9019) (-430.8685, -166.7624) (-423.3796, -161.6792) (-418.5714, -160.7174) knots 0 0 0 0 1 1 1 1
  spline S25 degree 3 poles (-418.5714, -160.7174) (-416.0694, -160.217) (-412.4596, -157.459) (-407.6974, -152.4097) knots 0 0 0 0 1 1 1 1
  spline S26 degree 3 poles (-407.6974, -152.4097) (-403.7766, -148.2524) (-399.8472, -144.8513) (-398.9647, -144.8513) knots 0 0 0 0 1 1 1 1
  spline S27 degree 3 poles (-398.9647, -144.8513) (-397.6998, -144.8513) (-397.754, -144.2899) (-399.2212, -142.1953) knots 0 0 0 0 1 1 1 1
  spline S28 degree 3 poles (-399.2212, -142.1953) (-400.2443, -140.7345) (-401.0815, -138.2879) (-401.0815, -136.7584) knots 0 0 0 0 1 1 1 1
  spline S29 degree 3 poles (-401.0815, -136.7584) (-401.0815, -135.2288) (-401.9958, -132.2563) (-403.1133, -130.1526) knots 0 0 0 0 1 1 1 1
  spline S30 degree 3 poles (-403.1133, -130.1526) (-404.6599, -127.2412) (-405.2611, -122.3336) (-405.6314, -109.5978) knots 0 0 0 0 1 1 1 1
  spline S31 degree 3 poles (-405.6314, -109.5978) (-405.899, -100.3959) (-406.6629, -92.1961) (-407.329, -91.376) knots 0 0 0 0 1 1 1 1
  spline S32 degree 3 poles (-407.329, -91.376) (-407.9951, -90.5559) (-409.7681, -85.5329) (-411.269, -80.2141) knots 0 0 0 0 1 1 1 1
  spline S33 degree 3 poles (-411.269, -80.2141) (-414.078, -70.2597) (-413.7834, -64.3357) (-410.3748, -62.2295) knots 0 0 0 0 1 1 1 1
  spline S34 degree 3 poles (-410.3748, -62.2295) (-409.1757, -61.4884) (-409.1713, -60.9969) (-410.3529, -59.8152) knots 0 0 0 0 1 1 1 1
  spline S35 degree 3 poles (-410.3529, -59.8152) (-412.3844, -57.7837) (-412.2152, -54.6361) (-409.9744, -52.7766) knots 0 0 0 0 1 1 1 1
  spline S36 degree 3 poles (-409.9744, -52.7766) (-408.4269, -51.4923) (-407.2094, -51.6696) (-402.7721, -53.8254) knots 0 0 0 0 1 1 1 1
  spline S37 degree 3 poles (-402.7721, -53.8254) (-399.8352, -55.2522) (-396.995, -56.4196) (-396.4605, -56.4196) knots 0 0 0 0 1 1 1 1
  spline S38 degree 3 poles (-396.4605, -56.4196) (-395.926, -56.4196) (-394.7608, -54.2141) (-393.8711, -51.5183) knots 0 0 0 0 1 1 1 1
  spline S39 degree 3 poles (-393.8711, -51.5183) (-392.428, -47.1455) (-389.0192, -42.7421) (-384.1975, -39.0223) knots 0 0 0 0 1 1 1 1
  spline S40 degree 3 poles (-384.1975, -39.0223) (-379.0998, -35.0894) (-368.1026, -21.0773) (-366.89, -16.9696) knots 0 0 0 0 1 1 1 1
  spline S41 degree 3 poles (-366.89, -16.9696) (-365.4879, -12.2211) (-356.7068, -0.0605) (-350.5917, 5.601) knots 0 0 0 0 1 1 1 1
  spline S42 degree 3 poles (-350.5917, 5.601) (-348.7842, 7.2744) (-347.3054, 9.8682) (-347.3054, 11.3651) knots 0 0 0 0 1 1 1 1
  spline S43 degree 3 poles (-347.3054, 11.3651) (-347.3054, 13.2899) (-346.6058, 14.0865) (-344.9154, 14.0865) knots 0 0 0 0 1 1 1 1
  spline S44 degree 3 poles (-344.9154, 14.0865) (-343.5703, 14.0865) (-342.5254, 14.8832) (-342.5254, 15.9086) knots 0 0 0 0 1 1 1 1
  spline S45 degree 3 poles (-342.5254, 15.9086) (-342.5254, 19.4558) (-332.7886, 21.3748) (-329.0332, 18.5679) knots 0 0 0 0 1 1 1 1
  spline S46 degree 3 poles (-322.8096, -64.7452) (-323.4669, -65.2358) (-326.5477, -66.5881) (-329.6558, -67.7504) knots 0 0 0 0 1 1 1 1
  spline S47 degree 3 poles (-329.6558, -67.7504) (-332.7639, -68.9128) (-337.0362, -71.1394) (-339.1495, -72.6985) knots 0 0 0 0 1 1 1 1
  spline S48 degree 3 poles (-339.1495, -72.6985) (-341.2628, -74.2576) (-343.9388, -75.5333) (-345.0961, -75.5333) knots 0 0 0 0 1 1 1 1
  spline S49 degree 3 poles (-345.0961, -75.5333) (-347.5821, -75.5333) (-362.7421, -68.5136) (-365.0199, -66.3073) knots 0 0 0 0 1 1 1 1
  spline S50 degree 3 poles (-365.0199, -66.3073) (-369.832, -61.6467) (-374.5603, -68.447) (-373.7194, -78.8195) knots 0 0 0 0 1 1 1 1
  spline S51 degree 3 poles (-373.7194, -78.8195) (-373.5893, -80.4246) (-370.4737, -80.9013) (-369.8141, -79.4171) knots 0 0 0 0 1 1 1 1
  spline S52 degree 3 poles (-369.8141, -79.4171) (-369.595, -78.9241) (-366.9481, -77.36) (-363.9321, -75.9411) knots 0 0 0 0 1 1 1 1
  spline S53 degree 3 poles (-363.9321, -75.9411) (-355.8141, -72.1224) (-355.0753, -73.0985) (-355.0753, -87.6398) knots 0 0 0 0 1 1 1 1
  spline S54 degree 3 poles (-355.0753, -87.6398) (-355.0753, -99.9681) (-354.1072, -102.5467) (-350.5537, -99.6841) knots 0 0 0 0 1 1 1 1
  spline S55 degree 3 poles (-350.5537, -99.6841) (-349.7543, -99.04) (-344.2602, -95.8368) (-338.345, -92.5656) knots 0 0 0 0 1 1 1 1
  spline S56 degree 3 poles (-338.345, -92.5656) (-332.4297, -89.2945) (-325.8373, -84.9793) (-323.6954, -82.9764) knots 0 0 0 0 1 1 1 1
  spline S57 degree 3 poles (-323.6954, -82.9764) (-321.5535, -80.9736) (-316.8479, -77.6681) (-313.2386, -75.6312) knots 0 0 0 0 1 1 1 1
  spline S58 degree 3 poles (-313.2386, -75.6312) (-306.0084, -71.5505) (-305.2318, -69.4575) (-309.3317, -65.0938) knots 0 0 0 0 1 1 1 1
  spline S59 degree 3 poles (-309.3317, -65.0938) (-311.5923, -62.6875) (-312.7018, -62.3855) (-316.8004, -63.0606) knots 0 0 0 0 1 1 1 1
  spline S60 degree 3 poles (-316.8004, -63.0606) (-319.4481, -63.4967) (-322.1521, -64.2549) (-322.8094, -64.7455) knots 0 0 0 0 1 1 1 1
  line L91 (-322.8094, -64.7455) -> (-322.8096, -64.7452)
  spline S61 degree 3 poles (-364.0385, -85.26) (-364.0385, -86.6747) (-367.7052, -89.9597) (-373.2522, -93.5142) knots 0 0 0 0 1 1 1 1
  spline S62 degree 3 poles (-373.2522, -93.5142) (-376.3805, -95.519) (-377.5586, -95.7206) (-379.6391, -94.6071) knots 0 0 0 0 1 1 1 1
  spline S63 degree 3 poles (-379.6391, -94.6071) (-381.9765, -93.3561) (-382.1172, -93.4756) (-381.3187, -96.033) knots 0 0 0 0 1 1 1 1
  spline S64 degree 3 poles (-381.3187, -96.033) (-380.8394, -97.5683) (-379.913, -99.1676) (-379.2601, -99.5871) knots 0 0 0 0 1 1 1 1
  spline S65 degree 3 poles (-379.2601, -99.5871) (-378.6072, -100.0066) (-378.4147, -100.9026) (-378.8323, -101.5782) knots 0 0 0 0 1 1 1 1
  spline S66 degree 3 poles (-378.8323, -101.5782) (-379.2499, -102.2537) (-379.0346, -104.2713) (-378.354, -106.0615) knots 0 0 0 0 1 1 1 1
  spline S67 degree 3 poles (-378.354, -106.0615) (-376.8485, -110.0216) (-379.1088, -113.1312) (-384.2382, -114.1572) knots 0 0 0 0 1 1 1 1
  spline S68 degree 3 poles (-384.2382, -114.1572) (-389.3298, -115.1754) (-392.3756, -113.893) (-393.9618, -110.0632) knots 0 0 0 0 1 1 1 1
  spline S69 degree 3 poles (-393.9618, -110.0632) (-395.9962, -105.1512) (-397.1166, -105.7296) (-398.5548, -112.4342) knots 0 0 0 0 1 1 1 1
  spline S70 degree 3 poles (-398.5548, -112.4342) (-400.4467, -121.2546) (-397.8291, -135.2726) (-394.2901, -135.2727) knots 0 0 0 0 1 1 1 1
  spline S71 degree 3 poles (-394.2901, -135.2727) (-392.9566, -135.2728) (-392.7212, -136.1411) (-393.318, -138.8579) knots 0 0 0 0 1 1 1 1
  spline S72 degree 3 poles (-393.318, -138.8579) (-393.7511, -140.8296) (-393.6821, -142.443) (-393.1647, -142.443) knots 0 0 0 0 1 1 1 1
  spline S73 degree 3 poles (-393.1647, -142.443) (-391.8086, -142.443) (-383.16, -133.8081) (-383.1599, -132.4538) knots 0 0 0 0 1 1 1 1
  spline S74 degree 3 poles (-383.1599, -132.4538) (-383.1599, -131.3301) (-377.9236, -125.5921) (-365.4073, -112.9997) knots 0 0 0 0 1 1 1 1
  line L92 (-365.4073, -112.9997) -> (-359.0093, -106.5628)
  line L93 (-359.0093, -106.5628) -> (-359.8673, -95.5242)
  spline S75 degree 3 poles (-359.8673, -95.5242) (-360.3392, -89.4533) (-360.9705, -84.0738) (-361.2702, -83.5702) knots 0 0 0 0 1 1 1 1
  spline S76 degree 3 poles (-361.2702, -83.5702) (-361.9723, -82.3901) (-364.04, -83.6524) (-364.04, -85.2611) knots 0 0 0 0 1 1 1 1
  line L94 (-364.04, -85.2611) -> (-364.0385, -85.26)
  spline S77 degree 3 poles (-69.9128, -57.1685) (-70.176, -57.7898) (-70.3353, -58.7343) (-70.2669, -59.2672) knots 0 0 0 0 1 1 1 1
  spline S78 degree 3 poles (-66.1098, -45.5661) (-72.7999, -42.6775) (-79.68, -40.6969) (-84.3741, -40.3079) knots 0 0 0 0 1 1 1 1
  spline S79 degree 3 poles (-62.4815, -87.7805) (-60.4144, -80.6836) (-58.6819, -56.2234) (-59.8595, -50.7648) knots 0 0 0 0 1 1 1 1
  spline S80 degree 3 poles (-71.6834, -54.5969) (-69.8327, -55.7835) (-69.5192, -56.239) (-69.9128, -57.1685) knots 0 0 0 0 1 1 1 1
  spline S81 degree 3 poles (-59.8595, -50.7648) (-60.45, -48.0282) (-60.4959, -47.9901) (-66.1098, -45.5661) knots 0 0 0 0 1 1 1 1
  spline S82 degree 3 poles (-76.5096, -114.6411) (-76.1157, -115.7233) (-75.6688, -115.8539) (-74.1947, -115.3174) knots 0 0 0 0 1 1 1 1
  spline S83 degree 3 poles (-129.0308, -135.166) (-127.3423, -133.7459) (-127.582, -132.679) (-130.5025, -128.6131) knots 0 0 0 0 1 1 1 1
  spline S84 degree 3 poles (-178.2865, -15.3701) (-178.5334, -14.7718) (-178.926, -14.524) (-179.1592, -14.8194) knots 0 0 0 0 1 1 1 1
  spline S85 degree 3 poles (-148.9598, -53.1145) (-150.8779, -46.6854) (-153.7349, -39.6687) (-154.7919, -33.624) knots 0 0 0 0 1 1 1 1
  line L95 (-188.7399, -0.7287) -> (-189.0051, 0)
  spline S86 degree 3 poles (-82.3142, -96.0317) (-80.8591, -97.1801) (-81.4531, -105.6318) (-83.0888, -107.0535) knots 0 0 0 0 1 1 1 1
  spline S87 degree 3 poles (-121.2068, -143.1427) (-121.1966, -142.549) (-121.9202, -141.7328) (-122.8353, -141.3061) knots 0 0 0 0 1 1 1 1
  spline S88 degree 3 poles (-79.4365, -211.2784) (-81.2221, -208.1253) (-83.5633, -204.6981) (-84.6389, -203.663) knots 0 0 0 0 1 1 1 1
  spline S89 degree 3 poles (-103.0249, -32.4507) (-103.3722, -32.5771) (-103.4148, -32.8712) (-103.1195, -33.1042) knots 0 0 0 0 1 1 1 1
  spline S90 degree 3 poles (-186.5872, -3.0015) (-187.4809, -2.7423) (-188.3354, -1.8401) (-188.7399, -0.7287) knots 0 0 0 0 1 1 1 1
  spline S91 degree 3 poles (-70.2669, -59.2672) (-70.3926, -60.9836) (-70.8659, -62.7082) (-70.9678, -64.1804) knots 0 0 0 0 1 1 1 1
  spline S92 degree 3 poles (-162.7786, -20.375) (-166.2731, -21.3325) (-168.0229, -21.4708) (-169.6944, -20.9217) knots 0 0 0 0 1 1 1 1
  spline S93 degree 3 poles (-122.8353, -141.3061) (-123.7411, -140.8837) (-124.6215, -140.1553) (-124.7918, -139.6875) knots 0 0 0 0 1 1 1 1
  spline S94 degree 3 poles (-152.0887, -28.0582) (-151.7288, -27.6023) (-151.9309, -27.195) (-152.7563, -26.7125) knots 0 0 0 0 1 1 1 1
  spline S95 degree 3 poles (-132.5628, -84.676) (-130.6273, -86.7309) (-125.8288, -89.0335) (-121.5387, -89.9657) knots 0 0 0 0 1 1 1 1
  spline S96 degree 3 poles (-153.5956, -30.9793) (-152.7208, -30.838) (-152.0912, -30.4856) (-152.1965, -30.1964) knots 0 0 0 0 1 1 1 1
  line L96 (-145.0725, -76.8727) -> (-139.6588, -79.8807)
  spline S97 degree 3 poles (-152.1965, -30.1964) (-152.6058, -29.0718) (-152.5865, -28.6889) (-152.0887, -28.0582) knots 0 0 0 0 1 1 1 1
  spline S98 degree 3 poles (-129.4007, -136.0498) (-130.085, -136.2645) (-129.9482, -135.9374) (-129.0308, -135.166) knots 0 0 0 0 1 1 1 1
  spline S99 degree 3 poles (-87.2116, -23.5478) (-88.988, -25.1857) (-89.0133, -25.1867) (-89.5753, -23.6426) knots 0 0 0 0 1 1 1 1
  spline S100 degree 3 poles (-89.5753, -23.6426) (-91.0986, -20.9242) (-96.5777, -20.042) (-99.4834, -22.2152) knots 0 0 0 0 1 1 1 1
  spline S101 degree 3 poles (-128.3872, -72.8102) (-129.4627, -71.613) (-134.1338, -70.2563) (-133.2081, -68.992) knots 0 0 0 0 1 1 1 1
  spline S102 degree 3 poles (-71.1607, -115.5962) (-70.4967, -116.1152) (-69.7314, -116.4591) (-69.4601, -116.3603) knots 0 0 0 0 1 1 1 1
  spline S103 degree 3 poles (-107.0516, -33.9408) (-106.7842, -33.83) (-106.9049, -33.4739) (-107.3197, -33.1494) knots 0 0 0 0 1 1 1 1
  spline S104 degree 3 poles (-92.0911, -45.0244) (-85.2571, -44.0629) (-76.1399, -51.6985) (-71.6837, -54.5973) knots 0 0 0 0 1 1 1 1
  spline S105 degree 3 poles (-66.31, -116.4471) (-58.7633, -116.1747) (-54.7735, -110.4959) (-53.9972, -105.1142) knots 0 0 0 0 1 1 1 1
  spline S106 degree 3 poles (-102.1257, -161.073) (-103.2216, -160.6969) (-104.2696, -159.9735) (-104.4545, -159.4656) knots 0 0 0 0 1 1 1 1
  spline S107 degree 3 poles (-162.8988, -54.2456) (-163.3963, -54.4266) (-164.1374, -52.646) (-165.5322, -47.9185) knots 0 0 0 0 1 1 1 1
  spline S108 degree 3 poles (-152.7563, -26.7125) (-153.7036, -26.1588) (-153.9953, -26.2199) (-154.2165, -27.0184) knots 0 0 0 0 1 1 1 1